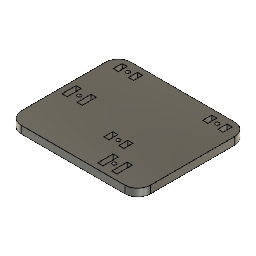
base v3 (Autodesk Fusion 360 design; units mm, degrees)
Autodesk Fusion 360 part; units mm, degrees
note: some values were not read from the file. Set by a fixed rule: which sketch regions a step uses.
sketch "Sketch1" plane through (0, 0, 0) normal (0, 0, 1) x (1, 0, 0)
  line L0 (10, 0) -> (91, 0)
  line L1 (101, 10) -> (101, 75.843)
  line L2 (91, 85.843) -> (10, 85.843)
  line L3 (0, 75.843) -> (0, 10)
  line L4 (8, 80.843) -> (23, 80.843)
  line L5 (23, 80.843) -> (23, 74.843)
  line L6 (23, 74.843) -> (8, 74.843)
  line L7 (8, 74.843) -> (8, 80.843)
  line L8 (23, 80.843) -> (78, 80.843)
  line L9 (78, 80.843) -> (93, 80.843)
  line L10 (93, 80.843) -> (93, 74.843)
  line L11 (93, 74.843) -> (78, 74.843)
  line L12 (78, 74.843) -> (78, 80.843)
  line L13 (11, 80.843) -> (11, 74.843)
  line L14 (20, 80.843) -> (20, 74.843)
  line L15 (90, 80.843) -> (90, 74.843)
  line L16 (81, 74.843) -> (81, 80.843)
  line L17 (50.5, 85.843) -> (50.5, 80.843)
  line L18 (5, 47.843) -> (19.74, 47.843)
  line L19 (19.74, 47.843) -> (19.74, 37.843)
  line L20 (19.74, 37.843) -> (5, 37.843)
  line L21 (5, 37.843) -> (5, 47.843)
  line L22 (5, 47.843) -> (8, 47.843)
  line L23 (8, 47.843) -> (8, 37.843)
  line L24 (8, 37.843) -> (5, 37.843)
  line L25 (5, 37.843) -> (5, 47.843)
  line L26 (19.74, 37.843) -> (16.74, 37.843)
  line L27 (16.74, 37.843) -> (16.74, 47.843)
  line L28 (16.74, 47.843) -> (19.74, 47.843)
  line L29 (19.74, 47.843) -> (19.74, 37.843)
  line L30 (50.557, 31) -> (65.297, 31)
  line L31 (65.297, 31) -> (65.297, 25)
  line L32 (65.297, 25) -> (50.557, 25)
  line L33 (50.557, 25) -> (50.557, 31)
  line L34 (50.557, 31) -> (53.557, 31)
  line L35 (53.557, 31) -> (53.557, 25)
  line L36 (53.557, 25) -> (50.557, 25)
  line L37 (50.557, 25) -> (50.557, 31)
  line L38 (65.297, 25) -> (62.297, 25)
  line L39 (62.297, 25) -> (62.297, 31)
  line L40 (62.297, 31) -> (65.297, 31)
  line L41 (65.297, 31) -> (65.297, 25)
  line L42 (65.797, 16) -> (79.797, 16)
  line L43 (79.797, 16) -> (79.797, 5)
  line L44 (79.797, 5) -> (65.797, 5)
  line L45 (65.797, 5) -> (65.797, 16)
  line L46 (68.797, 16) -> (68.797, 5)
  line L47 (76.797, 5) -> (76.797, 16)
  arc A0 (10, 85.843) -> (0, 75.843) centre (10, 75.843) ccw
  arc A1 (101, 75.843) -> (91, 85.843) centre (91, 75.843) ccw
  arc A2 (0, 10) -> (10, 0) centre (10, 10) ccw
  arc A3 (91, 0) -> (101, 10) centre (91, 10) ccw
  line L48 (11, 77.843) -> (20, 77.843)
  line L49 (8, 42.843) -> (16.74, 42.843)
  line L50 (81, 77.843) -> (90, 77.843)
  line L51 (53.557, 28) -> (62.297, 28)
  line L52 (68.797, 10.5) -> (76.797, 10.5)
  circle A4 centre (72.297, 10.5) radius 1.5
  circle A5 centre (57.927, 28) radius 1.5
  circle A6 centre (12.37, 42.843) radius 1.5
  circle A7 centre (15.5, 77.843) radius 1.5
  circle A8 centre (85.5, 77.843) radius 1.5
  circle A9 centre (72.297, 10.5) radius 3.5
  dimension "d1" = 6
  dimension "d2" = 6
  dimension "d3" = 15
  dimension "d4" = 15
  dimension "d5" = 55
  dimension "d6" = 3
  dimension "d7" = 3
  dimension "d8" = 3
  dimension "d9" = 3
  dimension "d10" = 90
  dimension "d11" = 5
  dimension "d12" = 14.74
  dimension "d13" = 10
  dimension "d14" = 3
  dimension "d15" = 3
  dimension "d16" = 27
  dimension "d17" = 3
  dimension "d18" = 14.74
  dimension "d19" = 6
  dimension "d20" = 3
  dimension "d21" = 3
  dimension "d22" = 6.843
  dimension "d23" = 30.817
  dimension "d24" = 14
  dimension "d25" = 11
  dimension "d26" = 3
  dimension "d27" = 3
  dimension "d28" = 0.5
  dimension "d29" = 9
  dimension "d30" = 5
  dimension "d31" = 8
  dimension "d32" = 8
  dimension "d33" = 5
  dimension "d34" = 10
  dimension "d35" = 10
  dimension "d36" = 10
  dimension "d37" = 10
  dimension "d38" = 7
  dimension "d39" = 3
  dimension "d40" = 3
  dimension "d41" = 3
  dimension "d42" = 3
  dimension "d43" = 3
  constraint horizontal L0
  constraint vertical L1
  constraint horizontal L2
  constraint vertical L3
  constraint horizontal L4
  constraint vertical L5
  constraint horizontal L6
  constraint vertical L7
  constraint perpendicular L5 L8
  constraint horizontal L9
  constraint vertical L10
  constraint horizontal L11
  constraint vertical L12
  constraint coincident L4 L13.start
  constraint coincident L6 L13.end
  constraint perpendicular L6 L13
  constraint coincident L4 L14.start
  constraint coincident L6 L14.end
  constraint perpendicular L6 L14
  constraint coincident L9 L15.start
  constraint coincident L11 L15.end
  constraint perpendicular L11 L15
  constraint coincident L11 L16.start
  constraint coincident L9 L16.end
  constraint perpendicular L9 L16
  constraint midpoint L8 L17.end
  constraint horizontal L18
  constraint vertical L19
  constraint horizontal L20
  constraint vertical L21
  constraint horizontal L22
  constraint vertical L23
  constraint horizontal L24
  constraint vertical L25
  constraint coincident L20 L23.end
  constraint horizontal L26
  constraint vertical L27
  constraint horizontal L28
  constraint vertical L29
  constraint coincident L18 L27.end
  constraint horizontal L30
  constraint vertical L31
  constraint horizontal L32
  constraint vertical L33
  constraint horizontal L34
  constraint vertical L35
  constraint horizontal L36
  constraint vertical L37
  constraint coincident L32 L35.end
  constraint horizontal L38
  constraint vertical L39
  constraint horizontal L40
  constraint vertical L41
  constraint horizontal L42
  constraint vertical L43
  constraint horizontal L44
  constraint vertical L45
  constraint coincident L42 L46.start
  constraint coincident L44 L46.end
  constraint perpendicular L44 L46
  constraint coincident L44 L47.start
  constraint coincident L42 L47.end
  constraint perpendicular L42 L47
  constraint coincident L2 L17.start
  constraint tangent L2 A0
  constraint tangent L3 A0
  constraint tangent L1 A1
  constraint tangent L2 A1
  constraint tangent L0 A2
  constraint tangent L3 A2
  constraint tangent L0 A3
  constraint tangent L1 A3
  constraint midpoint L13 L48.start
  constraint midpoint L14 L48.end
  constraint midpoint L23 L49.start
  constraint midpoint L27 L49.end
  constraint midpoint L16 L50.start
  constraint midpoint L15 L50.end
  constraint coincident L30 L39.end
  constraint midpoint L35 L51.start
  constraint midpoint L39 L51.end
  constraint midpoint L46 L52.start
  constraint midpoint L47 L52.end
  constraint midpoint L51 A5.centre
  constraint midpoint L49 A6.centre
  constraint midpoint L48 A7.centre
  constraint midpoint L50 A8.centre
  constraint coincident L52 A4.centre
  constraint concentric A4 A9
  constraint tangent L46 A9
  measures "d1" distance of L4.start L6.end
  measures "d2" distance of L9.end L10.end
  measures "d3" distance of L5.end L6.end
  measures "d4" distance of L10.end L11.end
  measures "d5" distance of L4.end L8.end
  measures "d6" distance of L12 L16
  measures "d7" distance of L10 L15
  measures "d8" distance of L7 L13
  measures "d9" distance of L5 L14
  measures "d10" angle of L2 L17
  measures "d11" distance of L17.start L17.end
  measures "d12" distance of L18.start L18.end
  measures "d13" distance of L18.start L20.end
  measures "d14" distance of L21 L23
  measures "d15" distance of L27 L29
  measures "d16" distance of L6 L18
  measures "d17" distance of L7 L25
  measures "d18" distance of L30.start L30.end
  measures "d19" distance of L30.start L32.end
  measures "d20" distance of L33 L35
  measures "d21" distance of L31 L39
  measures "d22" distance of L20 L30
  measures "d23" distance of L29 L33
  measures "d24" distance of L42.start L42.end
  measures "d25" distance of L42.end L43.end
  measures "d26" distance of L45 L46
  measures "d27" distance of L43 L47
  measures "d28" distance of L31 L45
  measures "d29" distance of L38 L42
  measures "d30" distance of L3 L21
  measures "d31" distance of L3 L7
  measures "d32" distance of L1 L10
  measures "d33" distance of L0 L44
  measures "d34" radius of A0
  measures "d35" radius of A1
  measures "d36" radius of A2
  measures "d37" radius of A3
  measures "d38" diameter of A9
  measures "d39" diameter of A4
  measures "d40" diameter of A5
  measures "d41" diameter of A6
  measures "d42" diameter of A7
  measures "d43" diameter of A8
extrude "Extrude1" add sketch "Sketch1" along normal blind 6 contours L0 L1 L2 L3 A0 A1 A2 A3 | L4 L13 L14 L48 A7 | L6 L13 L14 L48 A7 | L9 L15 L16 L50 A8 | L11 L15 L16 L50 A8 | L18 L23 L27 L49 A6 | L20 L23 L27 L49 A6 | L30 L35 L39 L51 A5 | L32 L35 L39 L51 A5 | L42 L46 L47 L52 A9 | L44 L46 L47 L52 A9 | L52 A4 A9 | L52 A4 A9
sketch "Sketch2" plane through (0, 0, 6) normal (0, 0, 1) x (-1, 0, 0)
  line L0 (-8, -80.843) -> (-11, -80.843)
  line L1 (-11, -80.843) -> (-11, -74.843)
  line L2 (-11, -74.843) -> (-8, -74.843)
  line L3 (-8, -74.843) -> (-8, -80.843)
  line L4 (-16.74, -47.843) -> (-19.74, -47.843)
  line L5 (-19.74, -47.843) -> (-19.74, -37.843)
  line L6 (-19.74, -37.843) -> (-16.74, -37.843)
  line L7 (-16.74, -37.843) -> (-16.74, -47.843)
  line L8 (-65.797, -16) -> (-68.797, -16)
  line L9 (-68.797, -16) -> (-68.797, -5)
  line L10 (-68.797, -5) -> (-65.797, -5)
  line L11 (-65.797, -5) -> (-65.797, -16)
  circle A0 centre (-57.927, -28) radius 1.5
  line L12 (-81, -74.843) -> (-78, -74.843)
  line L13 (-78, -74.843) -> (-78, -80.843)
  line L14 (-78, -80.843) -> (-81, -80.843)
  line L15 (-81, -80.843) -> (-81, -74.843)
  circle A1 centre (-85.5, -77.843) radius 1.5
  line L16 (-90, -80.843) -> (-93, -80.843)
  line L17 (-93, -80.843) -> (-93, -74.843)
  line L18 (-93, -74.843) -> (-90, -74.843)
  line L19 (-90, -74.843) -> (-90, -80.843)
  circle A2 centre (-15.5, -77.843) radius 1.5
  line L20 (-20, -80.843) -> (-23, -80.843)
  line L21 (-23, -80.843) -> (-23, -74.843)
  line L22 (-23, -74.843) -> (-20, -74.843)
  line L23 (-20, -74.843) -> (-20, -80.843)
  line L24 (-53.557, -25) -> (-50.557, -25)
  line L25 (-50.557, -25) -> (-50.557, -31)
  line L26 (-50.557, -31) -> (-53.557, -31)
  line L27 (-53.557, -31) -> (-53.557, -25)
  line L28 (-8, -37.843) -> (-5, -37.843)
  line L29 (-5, -37.843) -> (-5, -47.843)
  line L30 (-5, -47.843) -> (-8, -47.843)
  line L31 (-8, -47.843) -> (-8, -37.843)
  circle A3 centre (-72.297, -10.5) radius 1.5
  circle A4 centre (-12.37, -42.843) radius 1.5
  line L32 (-62.297, -31) -> (-65.297, -31)
  line L33 (-65.297, -31) -> (-65.297, -25)
  line L34 (-65.297, -25) -> (-62.297, -25)
  line L35 (-62.297, -25) -> (-62.297, -31)
  line L36 (-79.797, -5) -> (-76.797, -5)
  line L37 (-76.797, -5) -> (-76.797, -16)
  line L38 (-76.797, -16) -> (-79.797, -16)
  line L39 (-79.797, -16) -> (-79.797, -5)
  arc A5 (-91, 0) -> (-101, -10) centre (-91, -10) ccw
  line L40 (-101, -10) -> (-101, -75.843)
  arc A6 (-101, -75.843) -> (-91, -85.843) centre (-91, -75.843) ccw
  line L41 (-91, -85.843) -> (-10, -85.843)
  arc A7 (-10, -85.843) -> (0, -75.843) centre (-10, -75.843) ccw
  line L42 (0, -75.843) -> (0, -10)
  arc A8 (0, -10) -> (-10, 0) centre (-10, -10) ccw
  line L43 (-10, 0) -> (-91, 0)
  line L44 (-7.5, -74.343) -> (-7.5, -81.343)
  line L45 (-7.5, -81.343) -> (-11.5, -81.343)
  line L46 (-11.5, -81.343) -> (-11.5, -74.343)
  line L47 (-11.5, -74.343) -> (-7.5, -74.343)
  line L48 (-23.5, -74.343) -> (-19.5, -74.343)
  line L49 (-19.5, -74.343) -> (-19.5, -81.343)
  line L50 (-19.5, -81.343) -> (-23.5, -81.343)
  line L51 (-23.5, -81.343) -> (-23.5, -74.343)
  line L52 (-81.5, -74.343) -> (-77.5, -74.343)
  line L53 (-77.5, -74.343) -> (-77.5, -81.343)
  line L54 (-77.5, -81.343) -> (-81.5, -81.343)
  line L55 (-81.5, -81.343) -> (-81.5, -74.343)
  line L56 (-93.5, -81.343) -> (-93.5, -74.343)
  line L57 (-93.5, -74.343) -> (-89.5, -74.343)
  line L58 (-89.5, -74.343) -> (-89.5, -81.343)
  line L59 (-89.5, -81.343) -> (-93.5, -81.343)
  line L60 (-4.5, -37.343) -> (-4.5, -48.343)
  line L61 (-4.5, -48.343) -> (-8.5, -48.343)
  line L62 (-8.5, -48.343) -> (-8.5, -37.343)
  line L63 (-8.5, -37.343) -> (-4.5, -37.343)
  line L64 (-20.24, -37.343) -> (-16.24, -37.343)
  line L65 (-16.24, -37.343) -> (-16.24, -48.343)
  line L66 (-16.24, -48.343) -> (-20.24, -48.343)
  line L67 (-20.24, -48.343) -> (-20.24, -37.343)
  line L68 (-50.057, -31.5) -> (-54.057, -31.5)
  line L69 (-54.057, -31.5) -> (-54.057, -24.5)
  line L70 (-54.057, -24.5) -> (-50.057, -24.5)
  line L71 (-50.057, -24.5) -> (-50.057, -31.5)
  line L72 (-61.797, -31.5) -> (-65.797, -31.5)
  line L73 (-65.797, -31.5) -> (-65.797, -24.5)
  line L74 (-65.797, -24.5) -> (-61.797, -24.5)
  line L75 (-61.797, -24.5) -> (-61.797, -31.5)
  line L76 (-69.297, -4.5) -> (-65.297, -4.5)
  line L77 (-65.297, -4.5) -> (-65.297, -16.5)
  line L78 (-65.297, -16.5) -> (-69.297, -16.5)
  line L79 (-69.297, -16.5) -> (-69.297, -4.5)
  line L80 (-80.297, -4.5) -> (-76.297, -4.5)
  line L81 (-76.297, -4.5) -> (-76.297, -16.5)
  line L82 (-76.297, -16.5) -> (-80.297, -16.5)
  line L83 (-80.297, -16.5) -> (-80.297, -4.5)
  dimension "d46" = -0.5
  dimension "d47" = -0.5
  dimension "d48" = -0.5
  dimension "d49" = -0.5
  dimension "d50" = -0.5
  dimension "d51" = -0.5
  dimension "d52" = -0.5
  dimension "d53" = -0.5
  dimension "d54" = -0.5
  dimension "d55" = -0.5
extrude "Extrude2" cut sketch "Sketch2" against normal blind 10 contours L44 L45 L46 L47 | L48 L49 L50 L51 | L52 L53 L54 L55 | L56 L57 L58 L59 | L60 L61 L62 L63 | L64 L65 L66 L67 | L68 L69 L70 L71 | L72 L73 L74 L75 | L76 L77 L78 L79 | L80 L81 L82 L83
